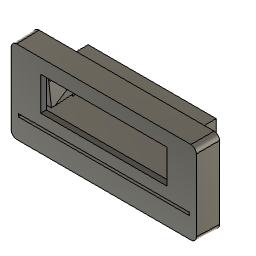
AmigaGotekEnclosure (Autodesk Fusion 360 design; units mm, degrees)
Autodesk Fusion 360 part; units mm, degrees
note: some values were not read from the file. Set by a fixed rule: which face or edge a step refers to.
sketch "Sketch1" plane through (0, 0, 0) normal (0, 1, 0) x (1, 0, 0) in component "face"
  line L0 (77.7875, 34.925) -> (-77.7875, 34.925)
  line L1 (-77.7875, 34.925) -> (-77.7875, -34.925)
  line L2 (-77.7875, -34.925) -> (77.7875, -34.925)
  line L3 (77.7875, -34.925) -> (77.7875, 34.925)
  line L4 (77.7875, 34.925) -> (-77.7875, -34.925) construction
  line L5 (-77.7875, 34.925) -> (77.7875, -34.925) construction
  dimension "d29" = 155.575
  dimension "d30" = 69.85
  constraint horizontal L0
  constraint perpendicular L0 L1
  constraint parallel L0 L2
  constraint parallel L1 L3
  constraint coincident L4 origin
  constraint coincident L5 origin
  measures "d29" distance of L1.end L2.end
  measures "d30" distance of L0.end L1.end
extrude "Extrude1" add sketch "Sketch1" against normal blind 19.05 draft -1 in component "face"
fillet "Fillet1" radius 4.572 4 edges at (-77.6212, -9.525, 34.7587) (77.6212, -9.525, 34.7587) (77.6212, -9.525, -34.7587) (-77.6212, -9.525, -34.7587) in component "face"
shell "Shell1" thickness 2.3813 removed faces 1 at (-24.4054, 0, -11.6417) in component "face"
sketch "Sketch2" plane through (0, -19.05, 0) normal (0, -1, 0) x (1, 0, 0) in component "face"
  ellipse E0 centre (-72.8823, -30.0198) end of major axis (-76.1162, -33.2537) minor radius 4.572 (-77.455, -30.0212) -> (-72.8837, -34.5925) ccw
  line L0 (-72.8837, -34.5925) -> (72.8837, -34.5925)
  ellipse E1 centre (72.8823, -30.0198) end of major axis (76.1162, -33.2537) minor radius 4.572 (72.8837, -34.5925) -> (77.455, -30.0212) ccw
  line L1 (77.455, -30.0212) -> (77.455, 30.0212)
  ellipse E2 centre (72.8823, 30.0198) end of major axis (76.1162, 33.2537) minor radius 4.572 (77.455, 30.0212) -> (72.8837, 34.5925) ccw
  line L2 (72.8837, 34.5925) -> (-72.8837, 34.5925)
  ellipse E3 centre (-72.8823, 30.0198) end of major axis (-76.1162, 33.2537) minor radius 4.572 (-72.8837, 34.5925) -> (-77.455, 30.0212) ccw
  line L3 (-77.455, 30.0212) -> (-77.455, -30.0212)
  line L4 (71.4375, -17.5269) -> (-71.4375, -17.5269)
  line L5 (-71.4375, -17.5269) -> (-71.4375, -15.1456)
  line L6 (-71.4375, -15.1456) -> (71.4375, -15.1456)
  line L7 (71.4375, -15.1456) -> (71.4375, -17.5269)
  line L8 (71.4375, -17.5269) -> (-71.4375, -15.1456) construction
  line L9 (-71.4375, -17.5269) -> (71.4375, -15.1456) construction
  line L10 (6.2218, -34.5925) -> (6.2218, -17.5269) construction
  point P0 (0, -16.3362)
  dimension "d36" = 142.875
  dimension "d37" = 2.3813
  dimension "d38" = 17.0656
  constraint horizontal L4
  constraint perpendicular L4 L5
  constraint parallel L4 L6
  constraint parallel L5 L7
  constraint coincident L8 P0
  constraint coincident L9 P0
  constraint coincident L0 L10.start
  constraint coincident L4 L10.end
  constraint perpendicular L4 L10
  measures "d36" distance of L5.end L6.end
  measures "d37" distance of L4.end L5.end
  measures "d38" distance of L10.start L10.end
extrude "Extrude2" cut sketch "Sketch2" against normal up to surface (2.3813 mm away) contours L4 L5 L6 L7 in component "face"
sketch "Sketch3" plane through (0, -16.6688, 0) normal (0, 1, 0) x (-1, 0, 0) in component "face"
  line L0 (-71.4375, -17.5269) -> (-71.4375, -15.1456)
  line L1 (-71.4375, -15.1456) -> (71.4375, -15.1456)
  line L2 (71.4375, -15.1456) -> (71.4375, -17.5269)
  line L3 (71.4375, -17.5269) -> (-71.4375, -17.5269)
  ellipse E0 centre (72.9238, -30.0613) end of major axis (74.4734, -31.6109) minor radius 2.1907 (72.9245, -32.2524) -> (75.1149, -30.062) ccw
  line L4 (75.1149, -30.062) -> (75.1149, 30.062)
  ellipse E1 centre (72.9238, 30.0613) end of major axis (74.4734, 31.6109) minor radius 2.1907 (75.1149, 30.062) -> (72.9245, 32.2524) ccw
  line L5 (72.9245, 32.2524) -> (-72.9245, 32.2524)
  ellipse E2 centre (-72.9238, 30.0613) end of major axis (-74.4734, 31.6109) minor radius 2.1907 (-72.9245, 32.2524) -> (-75.1149, 30.062) ccw
  line L6 (-75.1149, 30.062) -> (-75.1149, -30.062)
  ellipse E3 centre (-72.9238, -30.0613) end of major axis (-74.4734, -31.6109) minor radius 2.1907 (-75.1149, -30.062) -> (-72.9245, -32.2524) ccw
  line L7 (-72.9245, -32.2524) -> (72.9245, -32.2524)
  line L8 (0, -15.1456) -> (0, 32.2524) construction
  line L9 (53.5622, -6.3294) -> (-53.5622, -6.3294)
  line L10 (-53.5622, -6.3294) -> (-53.5622, 23.4362)
  line L11 (-53.5622, 23.4362) -> (53.5623, 23.4362)
  line L12 (53.5623, 23.4362) -> (53.5622, -6.3294)
  line L13 (53.5622, -6.3294) -> (-53.5622, 23.4362) construction
  line L14 (-53.5622, -6.3294) -> (53.5623, 23.4362) construction
  point P0 (0, 8.5534)
  dimension "d42" = 107.1245
  dimension "d43" = 29.7656
  constraint midpoint L1 L8.start
  constraint midpoint L5 L8.end
  constraint horizontal L9
  constraint perpendicular L9 L10
  constraint parallel L9 L11
  constraint parallel L10 L12
  constraint coincident L13 P0
  constraint coincident L14 P0
  constraint midpoint L8 P0
  measures "d42" distance of L10.end L11.end
  measures "d43" distance of L9.end L10.end
extrude "Extrude3" add sketch "Sketch3" along normal blind 38.1 contours L9 L10 L11 L12 in component "face"
shell "Shell2" thickness 2.3813 removed faces 1 at (-17.8541, 21.4312, 13.5144) in component "face"
ref_plane "WorkPlane4" through (53.5622, 2.3812, 8.5534) normal (1, 0, 0) x (0, 0, -1) in component "face"
sketch "Sketch8" plane through (53.5622, 0, 0) normal (1, 0, 0) x (0, 1, 0) in component "face"
  line L0 (-16.6688, 23.4362) -> (-16.6688, -6.3294)
  line L1 (-16.6688, -6.3294) -> (-16.6688, 23.4362)
  line L2 (-16.6688, -17.5269) -> (-16.6688, -15.1456)
  line L3 (-16.6688, -15.1456) -> (-16.6688, -17.5269)
  line L4 (-16.6688, -32.2524) -> (-16.6688, -30.062)
  line L5 (-16.6688, -30.062) -> (-16.6688, 30.062)
  line L6 (-16.6688, 30.062) -> (-16.6688, 32.2524)
  line L7 (-16.6688, 30.062) -> (-16.6688, 32.2524)
  line L8 (-16.6688, 30.062) -> (-16.6688, -30.062)
  line L9 (-16.6688, -32.2524) -> (-16.6688, -30.062)
  line L10 (-16.6688, -3.9481) -> (21.4312, -3.9481)
  line L11 (21.4312, -3.9481) -> (-16.6688, -3.9481)
  line L12 (-16.6688, 21.055) -> (21.4312, 21.055)
  line L13 (21.4312, 21.055) -> (-16.6688, 21.055)
  line L14 (-16.6688, 21.055) -> (-13.8906, 21.055)
  line L15 (-13.8906, 21.055) -> (-13.8906, -3.9481)
  line L16 (-13.8906, -3.9481) -> (-16.6688, -3.9481)
  line L17 (-16.6688, -3.9481) -> (-16.6688, 21.055)
  dimension "d60" = 2.7781
  constraint horizontal L14
  constraint vertical L15
  constraint horizontal L16
  constraint vertical L17
  constraint coincident L12.start L13.end
  measures "d60" distance of L12.start L14.end
extrude "Extrude6" cut sketch "Sketch8" against normal up to surface (107.1245 mm away) in component "face"
ref_plane "WorkPlane5" through (0, 2.3812, -3.9481) normal (0, 0, 1) x (1, 0, 0) in component "face"
sketch "Sketch9" plane through (0, 0, -3.9481) normal (0, 0, 1) x (1, 0, 0) in component "face"
  line L0 (-51.181, -13.8906) -> (-51.181, 21.4312) construction
  line L1 (-51.181, 21.4312) -> (-51.181, -13.8906) construction
  line L2 (51.181, -13.8906) -> (51.181, 21.4312) construction
  line L3 (51.181, 21.4312) -> (51.181, -13.8906) construction
  line L4 (-51.181, -13.8906) -> (51.181, -13.8906) construction
  line L5 (0, -13.8906) -> (0, 16.5449) construction
  line L6 (-51.181, -13.8906) -> (-48.7998, -13.8906)
  line L7 (-48.7998, -13.8906) -> (-51.181, 21.4312)
  line L8 (-51.181, 21.4312) -> (-51.181, -13.8906)
  line L9 (51.181, -13.8906) -> (48.7997, -13.8906)
  line L10 (48.7998, -13.8906) -> (51.181, 21.4313)
  line L11 (51.181, 21.4313) -> (51.181, -13.8906)
  dimension "d64" = 2.3813
  constraint coincident L0.start L1.end
  constraint coincident L2.start L3.end
  constraint midpoint L4 L5.start
  constraint perpendicular L4 L5
  constraint perpendicular L0 L6
  constraint coincident L0.end L1.start
  constraint symmetric L5 L0.start L2.start
  constraint symmetric L5 L6.end L10.start
  constraint symmetric L5 L0.end L10.end
  measures "d64" distance of L0.start L6.end
extrude "Extrude7" add sketch "Sketch9" along normal up to surface (25.0031 mm away) in component "face"
ref_plane "WorkPlane6" through (-51.181, -13.8906, 8.5534) normal (0, -1, 0) x (0, 0, 1) in component "face"
sketch "Sketch10" plane through (0, -13.8906, 0) normal (0, -1, 0) x (-1, 0, 0) in component "face"
  line L0 (51.181, -21.055) -> (48.7998, -21.055)
  line L1 (48.7998, -21.055) -> (48.7998, 3.9481)
  line L2 (48.7998, 3.9481) -> (51.181, 3.9481)
  line L3 (51.181, 3.9481) -> (51.181, -21.055)
  line L4 (-48.7998, -21.055) -> (-51.181, -21.055)
  line L5 (-51.181, -21.055) -> (-51.181, 3.9481)
  line L6 (-51.181, 3.9481) -> (-48.7997, 3.9481)
  line L7 (-48.7998, 3.9481) -> (-48.7998, -21.055)
  line L8 (51.181, 3.9481) -> (48.7998, 3.9481)
  line L9 (48.7998, 3.9481) -> (53.5623, 3.9481)
  line L10 (53.5623, 3.9481) -> (-53.5623, 3.9481)
  line L11 (-53.5623, 3.9481) -> (-48.7998, 3.9481)
  line L12 (-48.7998, 3.9481) -> (-51.181, 3.9481)
  line L13 (-51.181, 3.9481) -> (51.181, 3.9481)
  line L14 (48.7998, -21.055) -> (51.181, -21.055)
  line L15 (51.181, -21.055) -> (-51.181, -21.055)
  line L16 (-51.181, -21.055) -> (-48.7997, -21.055)
  line L17 (-48.7998, -21.055) -> (-53.5623, -21.055)
  line L18 (-53.5623, -21.055) -> (53.5623, -21.055)
  line L19 (53.5623, -21.055) -> (48.7998, -21.055)
  line L20 (53.5623, 3.9481) -> (53.5623, -21.055)
  line L21 (53.5623, -21.055) -> (53.5623, -23.4362)
  line L22 (53.5623, -23.4362) -> (53.5622, 6.3294)
  line L23 (53.5622, 6.3294) -> (53.5622, 3.9481)
  line L24 (-53.5622, -21.055) -> (-53.5622, 3.9481)
  line L25 (-53.5623, 3.9481) -> (-53.5622, 6.3294)
  line L26 (-53.5622, 6.3294) -> (-53.5622, -23.4362)
  line L27 (-53.5622, -23.4362) -> (-53.5622, -21.055)
  line L28 (48.7998, 3.9481) -> (-48.7998, 3.9481) construction
  line L29 (0, 3.9481) -> (0, -21.055) construction
  line L30 (51.181, 3.9481) -> (51.181, -15.4987) construction
  line L31 (51.181, -15.4987) -> (48.7998, 3.9481)
  line L32 (48.7998, 3.9481) -> (48.7998, -21.055)
  line L33 (48.7998, -21.055) -> (51.181, -21.055)
  line L34 (51.181, -21.055) -> (51.181, -15.4987)
  line L35 (-48.7998, -21.055) -> (-51.181, -21.055)
  line L36 (-48.7997, 3.9481) -> (-48.7998, -21.055)
  line L37 (-51.181, -21.055) -> (-51.181, -15.4987)
  line L38 (-51.181, -15.4987) -> (-48.7997, 3.9481)
  dimension "d68" = 19.4469
  constraint coincident L1.end L2.start
  constraint coincident L7.start L11.end
  constraint midpoint L28 L29.start
  constraint midpoint L18 L29.end
  constraint coincident L2.end L3.start
  constraint perpendicular L8 L30
  constraint coincident L0.end L1.start
  constraint coincident L0.start L3.end
  constraint symmetric L1.end L29 L6.end
  constraint symmetric L29 L30.end L37.end
  constraint symmetric L29 L1.end L6.end
  constraint symmetric L29 L0.end L4.start
  constraint symmetric L29 L0.start L4.end
  measures "d68" distance of L2.end L30.end
extrude "Extrude8" cut sketch "Sketch10" against normal up to surface (35.3219 mm away) contours L0 L1 L3 L14 L15 L18 L19 L31 L32 L33 L34 | L4 L5 L7 L15 L16 L17 L18 L35 L36 L37 L38 in component "face"
sketch "Sketch11" plane through (53.5622, 0, 0) normal (1, 0, 0) x (0, 1, 0) in component "face"
  line L0 (-16.6688, 21.055) -> (-13.8906, 21.055)
  line L1 (-13.8906, 21.055) -> (-13.8906, -3.9481)
  line L2 (-13.8906, -3.9481) -> (-16.6688, -3.9481)
  line L3 (-16.6688, -3.9481) -> (-16.6688, -6.3294)
  line L4 (-16.6688, -6.3294) -> (21.4312, -6.3294)
  line L5 (21.4312, -6.3294) -> (21.4312, 23.4362)
  line L6 (21.4312, 23.4362) -> (-16.6688, 23.4362)
  line L7 (-16.6688, 23.4362) -> (-16.6688, 21.055)
  line L8 (-13.8906, -3.9481) -> (21.4312, -3.9481)
  line L9 (21.4313, -3.9481) -> (-13.8906, -3.9481)
  line L10 (-13.8906, -3.9481) -> (-16.6687, -3.9481)
  line L11 (-16.6688, -3.9481) -> (-13.8906, -3.9481)
  line L12 (-13.8906, 21.055) -> (-13.8906, 15.4987)
  line L13 (-13.8906, 15.4987) -> (-13.8906, -3.9481)
  line L14 (-13.8906, -3.9481) -> (-13.8906, 21.055)
  line L15 (-13.8906, -3.9481) -> (5.1594, -3.9481)
  line L16 (5.1594, -3.9481) -> (5.1594, -2.3606)
  line L17 (5.1594, -2.3606) -> (-13.8906, -2.3606)
  line L18 (-13.8906, -2.3606) -> (-13.8906, -3.9481)
  dimension "d73" = 19.05
  dimension "d74" = 1.5875
  constraint horizontal L15
  constraint vertical L16
  constraint horizontal L17
  constraint vertical L18
  constraint coincident L1.end L2.start
  measures "d73" distance of L1.end L15.end
  measures "d74" distance of L1.end L17.end
extrude "Extrude9" cut sketch "Sketch11" against normal up to surface (107.1245 mm away) contours L1 L8 L9 L13 L14 L15 L16 L17 L18 in component "face"
ref_plane "WorkPlane7" through (0, -16.6688, 0) normal (0, 1, 0) x (1, 0, 0) in component "face"
sketch "Sketch14" plane through (0, -16.6688, 0) normal (0, 1, 0) x (1, 0, 0) in component "face"
  line L0 (51.181, -21.055) -> (51.181, -15.4987)
  line L1 (51.181, -15.4987) -> (51.181, -21.055)
  line L2 (51.181, -21.055) -> (53.5622, -21.055)
  line L3 (53.5623, -21.055) -> (-53.5623, -21.055)
  line L4 (-53.5623, -21.055) -> (-51.181, -21.055)
  line L5 (-51.181, -21.055) -> (51.181, -21.055)
  line L6 (-51.181, -15.4987) -> (-51.181, -21.055)
  line L7 (-51.181, -21.055) -> (-51.181, -15.4987)
  line L8 (50.084, 3.9481) -> (51.181, 3.9481)
  line L9 (51.181, 3.9481) -> (-51.181, 3.9481)
  line L10 (-51.181, 3.9481) -> (-50.084, 3.9481)
  line L11 (-50.084, 3.9481) -> (-53.5622, 3.9481)
  line L12 (-53.5622, 3.9481) -> (53.5623, 3.9481)
  line L13 (53.5623, 3.9481) -> (50.084, 3.9481)
  line L14 (51.181, -21.055) -> (-51.181, -21.055) construction
  line L15 (-51.181, -21.055) -> (-51.181, 3.9481) construction
  line L16 (-51.181, 3.9481) -> (51.181, 3.9481) construction
  line L17 (51.181, 3.9481) -> (51.181, -21.055) construction
  line L18 (-50.3872, -20.2612) -> (-50.3872, 3.1544)
  line L19 (-50.3872, 3.1544) -> (50.3872, 3.1544)
  line L20 (50.3873, 3.1544) -> (50.3872, -20.2612)
  line L21 (50.3872, -20.2612) -> (-50.3872, -20.2612)
  dimension "d81" = 0.7937
  constraint horizontal L14
  constraint vertical L15
  constraint horizontal L16
  constraint vertical L17
  constraint coincident L9.end L10.start
  constraint coincident L0.start L1.end
extrude "Extrude10" cut sketch "Sketch14" against normal up to surface (2.3812 mm away) in component "face"
ref_plane "WorkPlane8" through (0, 0, 0) normal (1, 0, 0) x (0, 1, 0) in component "face"
sketch "Sketch15" plane through (0, 0, 0) normal (1, 0, 0) x (0, 1, 0) in component "face"
  line L0 (-19.05, -3.1544) -> (-16.6688, -3.1544)
  line L1 (-16.6688, -3.1544) -> (-19.05, -3.1544)
  line L2 (-16.6688, 20.2612) -> (-16.6688, -3.1544)
  line L3 (-16.6688, -3.1544) -> (-16.6688, 20.2612)
  line L4 (-16.6688, -3.9481) -> (-16.6688, -6.3294)
  line L5 (-16.6688, -6.3294) -> (-16.6688, -3.9481)
  line L6 (-16.6688, -32.2524) -> (-16.6688, -30.062)
  line L7 (-16.6688, -30.062) -> (-16.6688, 30.062)
  line L8 (-16.6688, 30.062) -> (-16.6688, 32.2524)
  line L9 (-16.6688, 30.062) -> (-16.6688, 32.2524)
  line L10 (-16.6688, 30.062) -> (-16.6688, -30.062)
  line L11 (-16.6688, -32.2524) -> (-16.6688, -30.062)
  line L12 (-16.6688, -17.5269) -> (-16.6688, -15.1456)
  line L13 (-16.6688, -15.1456) -> (-16.6688, -17.5269)
  line L14 (-16.6688, 21.055) -> (-16.6688, 23.4362)
  line L15 (-16.6688, 23.4362) -> (-16.6688, 21.055)
  line L16 (-16.6688, -3.1544) -> (-19.05, -3.1544)
  line L17 (-19.05, -3.1544) -> (-19.05, -5.5356)
  line L18 (-19.05, -5.5356) -> (-16.6688, -3.1544)
  constraint coincident L0.end L1.start
  constraint coincident L0.start L1.end
  constraint perpendicular L1 L17
  constraint equal L16 L17
sweep "Sweep1" cut profiles "Sketch15" along 4 edges at (0, -16.6688, 20.2612) (-50.3872, -16.6688, 8.5534) (0, -16.6688, -3.1544) (50.3872, -16.6688, 8.5534) section 1 in component "face"
component "face" placed x (1, 0, 0) y (0, 1, 0) z (0, 0, 1) at (0, 0, 0)
equation "accent_line_bottom_offset = 43/64\"" comment "Face accent line distance from bottom"
equation "accent_line_height = 3/32\"" comment "Face accent line height"
equation "accent_line_width = enclosure_width - 1/2\"" comment "Face accent line height"
equation "enclosure_corner_radius = 0.18 in" comment "Corner radius for enclosure"
equation "enclosure_depth = 8 1/2\"" comment "Overall enclosure depth"
equation "enclosure_height = 2 3/4\"" comment "Overall enclosure height"
equation "enclosure_width = 6 1/8\"" comment "Overall enclosure width"
equation "face_depth = 3/4\"" comment "Face component depth"
equation "face_extrude_angle = 1 deg" comment "Face component extrude angle"
equation "gotek_mount_sleeve_depth = 1 1/2\"" comment "Gotek drive mounting sleeve depth"
equation "gotek_mount_sleeve_face_depth = 7/64\"" comment "Gotek drive face depth used to lock into mounting sleeve"
equation "gotek_mount_sleeve_height = 63/64\"" comment "Gotek drive mounting sleeve height"
equation "gotek_mount_sleeve_latch_height = 49/64\"" comment "Gotek drive mounting sleeve latch height"
equation "gotek_mount_sleeve_latch_width = 3/32\"" comment "Gotek drive mounting sleeve latch width"
equation "gotek_mount_sleeve_width = 4.03 in" comment "Gotek drive mounting sleeve width"
equation "shell_thickness = 3/32\"" comment "Overall enclosure shell thickness"
equation "d29 = enclosure_width"
equation "d30 = enclosure_height"
equation "d31 = -face_depth"
equation "d32 = -face_extrude_angle"
equation "d34 = enclosure_corner_radius"
equation "d35 = shell_thickness"
equation "d36 = accent_line_width"
equation "d37 = accent_line_height"
equation "d38 = accent_line_bottom_offset"
equation "d39 = 0\""
equation "accent_line_depth = 1/16\""
equation "d42 = gotek_mount_sleeve_width + ( shell_thickness * 2 )"
equation "d43 = gotek_mount_sleeve_height + ( shell_thickness * 2 )"
equation "d44 = gotek_mount_sleeve_depth"
equation "d46 = shell_thickness"
equation "d59 = 0\""
equation "d60 = gotek_mount_sleeve_face_depth"
equation "d61 = 0\""
equation "d63 = 0\""
equation "d64 = gotek_mount_sleeve_latch_width"
equation "d65 = 0\""
equation "d67 = 0\""
equation "d68 = gotek_mount_sleeve_latch_height"
equation "d69 = 0\""
equation "gotek_mounting_sleeve_latch_bottom_gap_height = 1/16\""
equation "gotek_mounting_sleeve_latch_bottom_gap_depth = gotek_mount_sleeve_depth * 0.5"
equation "d73 = gotek_mounting_sleeve_latch_bottom_gap_depth"
equation "d74 = gotek_mounting_sleeve_latch_bottom_gap_height"
equation "d75 = 0\""
equation "gotek_window_inset = 1/32\""
equation "d80 = 0\""
equation "d81 = gotek_window_inset"
equation "d82 = 0\""
equation "d84 = 0\""
named bodies: "face"
